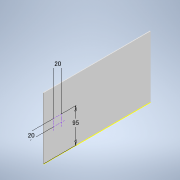
# Autodesk Inventor part: アーム支え
Saved by Autodesk Inventor 2022 (Build 260153000, 153)
## iProperties
Created: 2022-11-22
Part Number: アーム支え
Material: 一般
Document SubType Name: Modeling
Designer: tdn82
Density: 1 g/cm^3
Appearance: 既定
Author: tdn82
Autodesk Inventor part; units mm, degrees
ref_plane "YZ Plane" through (0, 0, 0) normal (1, 0, 0) x (0, 1, 0)
ref_plane "XZ Plane" through (0, 0, 0) normal (0, 1, 0) x (-1, 0, 0)
ref_plane "XY Plane" through (0, 0, 0) normal (0, 0, 1) x (1, 0, 0)
sketch "スケッチ1" plane through (0, 0, 0) normal (0, 1, 0) x (-1, 0, 0)
  line L0 (0, 0) -> (-2, 0)
  line L1 (-2, 0) -> (-2, -296)
  line L2 (-2, -296) -> (0, -296)
  line L3 (0, -296) -> (0, 0)
  dimension "d0" = 2
  dimension "d1" = 296
  constraints: 8 end point, 2 parallel, 1 horizontal, 1 perpendicular
  measures "d0" distance of L0.start L0.end
  measures "d1" distance of L2.end L0.start
extrude "押し出し1" add sketch "スケッチ1" along normal blind 170
sketch "スケッチ2" plane through (2, 0, 0) normal (1, 0, 0) x (0, 0, -1)
  line L0 (0, 0) -> (296, 0) projected
  point P0 (48.6919, 95)
  point P1 (28.6919, 95)
  point P2 (28.6919, 75)
  point P3 (48.6919, 75)
  dimension "d5" = 95
  dimension "d6" = 20
  dimension "d7" = 20
  measures "d5" distance from line of point (48.692, 95) L0
  measures "d6" distance of point (28.692, 95) point (48.692, 95)
  measures "d7" distance of point (28.692, 75) point (28.692, 95)
hole "穴1" at (2, 95, -48.6919) at (2, 95, -28.6919) at (2, 75, -28.6919) at (2, 75, -48.6919) direction (-1, 0, 0) diameter 3.5 end through all
